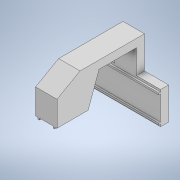
# Autodesk Inventor part: base
Saved by Autodesk Inventor 2020 (Build 240168000, 168)
## iProperties
Created: 2020-05-02
Part Number: base
Material: Generic
Document SubType Name: Modeling
Designer: zhang
Density: 1 g/cm^3
Appearance: Default
Author: zhang
Autodesk Inventor part; units mm, degrees
ref_plane "YZ Plane" through (0, 0, 0) normal (1, 0, 0) x (0, 1, 0)
ref_plane "XZ Plane" through (0, 0, 0) normal (0, 1, 0) x (-1, 0, 0)
ref_plane "XY Plane" through (0, 0, 0) normal (0, 0, 1) x (1, 0, 0)
sketch "Sketch1" plane through (0, 0, 0) normal (1, 0, 0) x (0, 1, 0)
  line L0 (0, 9.8901) -> (0, -9.3874)
  line L1 (-150, -257) -> (150, -257)
  line L2 (150, -257) -> (150, -332)
  line L3 (150, -332) -> (-150, -332)
  line L4 (-150, -332) -> (-150, -257)
  point P0 (0, 0)
  dimension "d0" = 257
  dimension "d1" = 300
  dimension "d2" = 75
  constraints: 10 end point, 2 parallel, 2 vertical, 1 horizontal, 1 perpendicular, 1 other
  measures "d0" distance from line of L1 point (0, 0)
  measures "d1" distance of L2.end L3.end
  measures "d2" distance of L1.end L2.end
extrude "Extrusion1" add sketch "Sketch1" along normal mid plane 650
sketch "Sketch2" plane through (0, 0, 0) normal (1, 0, 0) x (0, 1, 0)
  line L0 (450, -332) -> (450, 268)
  line L1 (450, 268) -> (328.8182, 483)
  line L2 (295, 543) -> (95, 543) construction
  line L3 (95, 483) -> (95, 193)
  line L4 (95, 193) -> (375, 193) construction
  line L5 (375, 91.0981) -> (375, -257)
  line L6 (-150, -332) -> (150, -332) projected
  line L7 (150, -332) -> (150, -257) projected
  line L8 (150, -332) -> (450, -332)
  line L9 (150, -257) -> (-150, -257) projected
  line L10 (150, -332) -> (150, -257)
  line L11 (150, -257) -> (150, -332) projected
  line L12 (150, -257) -> (375, -257)
  line L13 (95, 193) -> (375, 91.0981)
  line L14 (328.8182, 483) -> (95, 483)
  point P0 (0, 0)
  dimension "d7" = 75
  dimension "d8" = 300
  dimension "d9" = 600
  dimension "d10" = 280
  dimension "d11" = 450
  dimension "d12" = 350
  dimension "d13" = 200
  dimension "d22" = 60
  constraints: 22 end point, 5 perpendicular, 2 horizontal
  measures "d7" distance between parallel lines of L0 L5
  measures "d8" distance of L6.end L0.start
  measures "d9" distance of L0.start L0.end
  measures "d10" distance of L3.end L4.end
  measures "d11" distance of L4.end L5.end
  measures "d12" distance of L2.end L3.end
  measures "d13" distance of L2.start L2.end
  measures "d22" distance between parallel lines of L2 L14
extrude "Extrusion2" add sketch "Sketch2" along normal mid plane 200
sketch "Sketch3" plane through (-325, 0, 0) normal (-1, 0, 0) x (0, 0, 1)
  line L0 (-257, 150) -> (-257, -150) projected
  line L1 (-241, 130) -> (-257, 130)
  line L2 (-257, 130) -> (-257, 114)
  line L3 (-257, 114) -> (-241, 114)
  line L4 (-241, 114) -> (-241, 130)
  line L5 (-257, 150) -> (-332, 150) projected
  line L6 (-111.2497, 0) -> (-314.6527, 0)
  line L7 (-241, -130) -> (-257, -130)
  line L8 (-257, -130) -> (-257, -114)
  line L9 (-257, -114) -> (-241, -114)
  line L10 (-241, -114) -> (-241, -130)
  point P0 (0, 0)
  dimension "d23" = 20
  dimension "d24" = 16
  dimension "d25" = 16
  constraints: 18 end point, 4 symmetric about line, 3 horizontal, 2 parallel, 1 perpendicular, 1 point on line
  measures "d23" distance between parallel lines of L5 L1
  measures "d24" distance of L3.end L1.start
  measures "d25" distance of L2.end L3.end
extrude "Extrusion3" add sketch "Sketch3" against normal up to surface (650 mm away)
sketch "Sketch4" plane through (-100, 95, 483) normal (0, 0, 1) x (1, 0, 0)
  line L0 (100, -95) -> (100, 134.7598)
  line L1 (0, 0) -> (200, 0) projected
  line L2 (20, 0) -> (36, 0)
  line L3 (36, 0) -> (36, -16)
  line L4 (36, -16) -> (20, -16)
  line L5 (20, -16) -> (20, 0)
  line L6 (0, 0) -> (0, 233.8182) projected
  line L7 (180, 0) -> (164, 0)
  line L8 (164, 0) -> (164, -16)
  line L9 (164, -16) -> (180, -16)
  line L10 (180, -16) -> (180, 0)
  point P0 (36, 0)
  dimension "d28" = 20
  dimension "d29" = 16
  dimension "d30" = 16
  constraints: 18 end point, 4 symmetric about line, 2 parallel, 1 horizontal, 1 perpendicular, 1 point on line, 1 vertical
  measures "d28" distance between parallel lines of L5 L6
  measures "d29" distance of L3.end L4.end
  measures "d30" distance of L2.end L3.end
extrude "Extrusion4" add sketch "Sketch4" against normal up to surface surface through (0, 95, 193) normal (0, -0.342, -0.9397)
body "Solid1"
